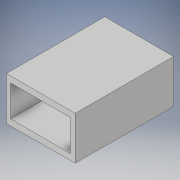
# Autodesk Inventor part: dc motor
Saved by Autodesk Inventor 2019 (Build 230136000, 136)
## iProperties
Created: 2019-12-08
Part Number: dc motor
Material: Generic
Document SubType Name: Modeling
Designer: HP
Density: 1 g/cm^3
Appearance: Default
Author: HP
Autodesk Inventor part; units mm, degrees
ref_plane "YZ Plane" through (0, 0, 0) normal (1, 0, 0) x (0, 1, 0)
ref_plane "XZ Plane" through (0, 0, 0) normal (0, 1, 0) x (-1, 0, 0)
ref_plane "XY Plane" through (0, 0, 0) normal (0, 0, 1) x (1, 0, 0)
sketch "Sketch1" plane through (0, 0, 0) normal (0, 0, 1) x (1, 0, 0)
  point P0 (0, 0)
sketch "Sketch2" plane through (0, 0, 0) normal (0, 0, 1) x (1, 0, 0)
  point P0 (0, 0)
sketch "Sketch3" plane through (0, 0, 0) normal (0, 0, 1) x (1, 0, 0)
  line L0 (0, 0) -> (7.112, 0)
  line L1 (7.112, 0) -> (7.112, 4.4704)
  line L2 (7.112, 4.4704) -> (0, 4.4704)
  line L3 (0, 4.4704) -> (0, 0)
  dimension "d0" = 7.112
  dimension "d1" = 4.4704
  constraints: 8 end point, 2 parallel, 1 horizontal, 1 perpendicular
  measures "d0" distance of L2.end L1.end
  measures "d1" distance of L1.end L0.end
extrude "Extrusion1" add sketch "Sketch3" along normal blind 10.16
sketch "Sketch4" plane through (0, 0, 10.16) normal (0, 0, 1) x (1, 0, 0)
  line L0 (0.4347, 3.8467) -> (6.6067, 3.8467)
  line L1 (6.6067, 3.8467) -> (6.6067, 0.6302)
  line L2 (6.6067, 0.6302) -> (0.4347, 0.6302)
  line L3 (0.4347, 0.6302) -> (0.4347, 3.8467)
  point P0 (0, 0)
  constraints: 8 end point, 2 parallel, 1 horizontal, 1 perpendicular
extrude "Extrusion2" cut sketch "Sketch4" against normal blind 7.62
sketch "Sketch5" plane through (0, 0, 0) normal (0, 0, -1) x (-1, 0, 0)
  circle A0 centre (-3.6638, 2.4113) radius 0.7685
  point P0 (0, 0)
  constraints: 1 centre point
extrude "Extrusion3" cut sketch "Sketch5" against normal blind 2.54
body "Solid1"
